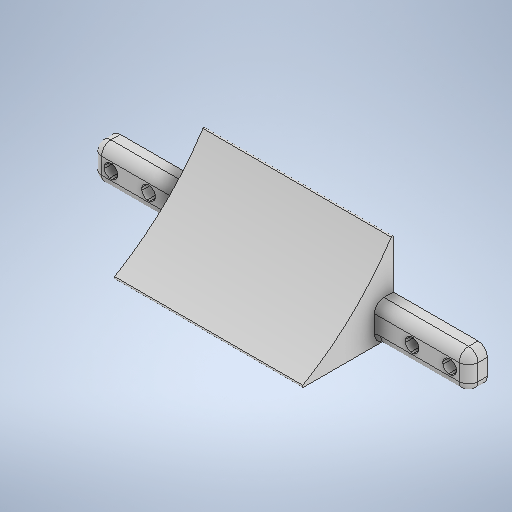
# Autodesk Inventor part: intake ramp piece
Saved by Autodesk Inventor 2025.1 (Build 291241020, 241B)
## iProperties
Created: 2024-12-04
Part Number: intake ramp piece
Material: Generic
Document SubType Name: Modeling
Designer: Hunter Mathis
Density: 1 g/cm^3
Appearance: Default
Author: Hunter Mathis
Autodesk Inventor part; units mm, degrees
ref_plane "YZ Plane" through (0, 0, 0) normal (1, 0, 0) x (0, 1, 0)
ref_plane "XZ Plane" through (0, 0, 0) normal (0, 1, 0) x (-1, 0, 0)
ref_plane "XY Plane" through (0, 0, 0) normal (0, 0, 1) x (1, 0, 0)
sketch "Sketch1" plane through (0, 0, 0) normal (0, 0, 1) x (1, 0, 0)
  line L0 (0, 0) -> (127, 0)
  line L1 (127, 0) -> (127, 11.9126)
  line L2 (127, 11.9126) -> (0, 11.9126)
  line L3 (0, 11.9126) -> (0, 0)
  dimension "d0" = 127
  dimension "d1" = 11.9126
  constraints: 8 end point, 2 parallel, 1 horizontal, 1 perpendicular
  measures "d0" distance of L1.end L2.end
  measures "d1" distance of L0.end L1.end
extrude "Extrusion1" add sketch "Sketch1" along normal blind 6.35
sketch "Sketch3" plane through (0, 0, 0) normal (0, 0, -1) x (-1, 0, 0)
  line L0 (-127, 0) -> (-127, 11.9126) projected
  line L1 (-127, 5.9563) -> (-120.65, 5.9563)
  line L2 (-127, 11.9126) -> (0, 11.9126) projected
  line L3 (0, 0) -> (-127, 0) projected
  line L4 (0, 11.9126) -> (0, 0) projected
  line L5 (-121.412, 8.2423) -> (-119.888, 8.2423)
  line L6 (-118.364, 6.7183) -> (-118.364, 5.1943)
  line L7 (-119.888, 3.6703) -> (-121.412, 3.6703)
  line L8 (-122.936, 5.1943) -> (-122.936, 6.7183)
  arc A0 (-121.412, 8.2423) -> (-122.936, 6.7183) centre (-121.412, 6.7183) ccw
  arc A1 (-118.364, 6.7183) -> (-119.888, 8.2423) centre (-119.888, 6.7183) ccw
  arc A2 (-119.888, 3.6703) -> (-118.364, 5.1943) centre (-119.888, 5.1943) ccw
  arc A3 (-122.936, 5.1943) -> (-121.412, 3.6703) centre (-121.412, 5.1943) ccw
  line L9 (-107.188, 3.6703) -> (-108.712, 3.6703)
  line L10 (-105.664, 6.7183) -> (-105.664, 5.1943)
  arc A4 (-105.664, 6.7183) -> (-107.188, 8.2423) centre (-107.188, 6.7183) ccw
  arc A5 (-110.236, 5.1943) -> (-108.712, 3.6703) centre (-108.712, 5.1943) ccw
  line L11 (-110.236, 5.1943) -> (-110.236, 6.7183)
  line L12 (-108.712, 8.2423) -> (-107.188, 8.2423)
  arc A6 (-108.712, 8.2423) -> (-110.236, 6.7183) centre (-108.712, 6.7183) ccw
  arc A7 (-107.188, 3.6703) -> (-105.664, 5.1943) centre (-107.188, 5.1943) ccw
  line L13 (-94.488, 3.6703) -> (-96.012, 3.6703)
  line L14 (-92.964, 6.7183) -> (-92.964, 5.1943)
  arc A8 (-92.964, 6.7183) -> (-94.488, 8.2423) centre (-94.488, 6.7183) ccw
  arc A9 (-97.536, 5.1943) -> (-96.012, 3.6703) centre (-96.012, 5.1943) ccw
  line L15 (-97.536, 5.1943) -> (-97.536, 6.7183)
  line L16 (-96.012, 8.2423) -> (-94.488, 8.2423)
  arc A10 (-96.012, 8.2423) -> (-97.536, 6.7183) centre (-96.012, 6.7183) ccw
  arc A11 (-94.488, 3.6703) -> (-92.964, 5.1943) centre (-94.488, 5.1943) ccw
  line L17 (-81.788, 3.6703) -> (-83.312, 3.6703)
  line L18 (-80.264, 6.7183) -> (-80.264, 5.1943)
  arc A12 (-80.264, 6.7183) -> (-81.788, 8.2423) centre (-81.788, 6.7183) ccw
  arc A13 (-84.836, 5.1943) -> (-83.312, 3.6703) centre (-83.312, 5.1943) ccw
  line L19 (-84.836, 5.1943) -> (-84.836, 6.7183)
  line L20 (-83.312, 8.2423) -> (-81.788, 8.2423)
  arc A14 (-83.312, 8.2423) -> (-84.836, 6.7183) centre (-83.312, 6.7183) ccw
  arc A15 (-81.788, 3.6703) -> (-80.264, 5.1943) centre (-81.788, 5.1943) ccw
  line L21 (-69.088, 3.6703) -> (-70.612, 3.6703)
  line L22 (-67.564, 6.7183) -> (-67.564, 5.1943)
  arc A16 (-67.564, 6.7183) -> (-69.088, 8.2423) centre (-69.088, 6.7183) ccw
  arc A17 (-72.136, 5.1943) -> (-70.612, 3.6703) centre (-70.612, 5.1943) ccw
  line L23 (-72.136, 5.1943) -> (-72.136, 6.7183)
  line L24 (-70.612, 8.2423) -> (-69.088, 8.2423)
  arc A18 (-70.612, 8.2423) -> (-72.136, 6.7183) centre (-70.612, 6.7183) ccw
  arc A19 (-69.088, 3.6703) -> (-67.564, 5.1943) centre (-69.088, 5.1943) ccw
  line L25 (-56.388, 3.6703) -> (-57.912, 3.6703)
  line L26 (-54.864, 6.7183) -> (-54.864, 5.1943)
  arc A20 (-54.864, 6.7183) -> (-56.388, 8.2423) centre (-56.388, 6.7183) ccw
  arc A21 (-59.436, 5.1943) -> (-57.912, 3.6703) centre (-57.912, 5.1943) ccw
  line L27 (-59.436, 5.1943) -> (-59.436, 6.7183)
  line L28 (-57.912, 8.2423) -> (-56.388, 8.2423)
  arc A22 (-57.912, 8.2423) -> (-59.436, 6.7183) centre (-57.912, 6.7183) ccw
  arc A23 (-56.388, 3.6703) -> (-54.864, 5.1943) centre (-56.388, 5.1943) ccw
  line L29 (-43.688, 3.6703) -> (-45.212, 3.6703)
  line L30 (-42.164, 6.7183) -> (-42.164, 5.1943)
  arc A24 (-42.164, 6.7183) -> (-43.688, 8.2423) centre (-43.688, 6.7183) ccw
  arc A25 (-46.736, 5.1943) -> (-45.212, 3.6703) centre (-45.212, 5.1943) ccw
  line L31 (-46.736, 5.1943) -> (-46.736, 6.7183)
  line L32 (-45.212, 8.2423) -> (-43.688, 8.2423)
  arc A26 (-45.212, 8.2423) -> (-46.736, 6.7183) centre (-45.212, 6.7183) ccw
  arc A27 (-43.688, 3.6703) -> (-42.164, 5.1943) centre (-43.688, 5.1943) ccw
  line L33 (-30.988, 3.6703) -> (-32.512, 3.6703)
  line L34 (-29.464, 6.7183) -> (-29.464, 5.1943)
  arc A28 (-29.464, 6.7183) -> (-30.988, 8.2423) centre (-30.988, 6.7183) ccw
  arc A29 (-34.036, 5.1943) -> (-32.512, 3.6703) centre (-32.512, 5.1943) ccw
  line L35 (-34.036, 5.1943) -> (-34.036, 6.7183)
  line L36 (-32.512, 8.2423) -> (-30.988, 8.2423)
  arc A30 (-32.512, 8.2423) -> (-34.036, 6.7183) centre (-32.512, 6.7183) ccw
  arc A31 (-30.988, 3.6703) -> (-29.464, 5.1943) centre (-30.988, 5.1943) ccw
  line L37 (-18.288, 3.6703) -> (-19.812, 3.6703)
  line L38 (-16.764, 6.7183) -> (-16.764, 5.1943)
  arc A32 (-16.764, 6.7183) -> (-18.288, 8.2423) centre (-18.288, 6.7183) ccw
  arc A33 (-21.336, 5.1943) -> (-19.812, 3.6703) centre (-19.812, 5.1943) ccw
  line L39 (-21.336, 5.1943) -> (-21.336, 6.7183)
  line L40 (-19.812, 8.2423) -> (-18.288, 8.2423)
  arc A34 (-19.812, 8.2423) -> (-21.336, 6.7183) centre (-19.812, 6.7183) ccw
  arc A35 (-18.288, 3.6703) -> (-16.764, 5.1943) centre (-18.288, 5.1943) ccw
  line L41 (-5.588, 3.6703) -> (-7.112, 3.6703)
  line L42 (-4.064, 6.7183) -> (-4.064, 5.1943)
  arc A36 (-4.064, 6.7183) -> (-5.588, 8.2423) centre (-5.588, 6.7183) ccw
  arc A37 (-8.636, 5.1943) -> (-7.112, 3.6703) centre (-7.112, 5.1943) ccw
  line L43 (-8.636, 5.1943) -> (-8.636, 6.7183)
  line L44 (-7.112, 8.2423) -> (-5.588, 8.2423)
  arc A38 (-7.112, 8.2423) -> (-8.636, 6.7183) centre (-7.112, 6.7183) ccw
  arc A39 (-5.588, 3.6703) -> (-4.064, 5.1943) centre (-5.588, 5.1943) ccw
  circle A40 centre (-120.65, 5.9563) radius 2.3241
  circle A41 centre (-107.95, 5.9563) radius 2.3241
  circle A42 centre (-19.05, 5.9563) radius 2.3241
  circle A43 centre (-6.35, 5.9563) radius 2.3241
  point P0 (-95.25, 5.9563)
  point P1 (-82.55, 5.9563)
  point P2 (-69.85, 5.9563)
  point P3 (-57.15, 5.9563)
  point P4 (-44.45, 5.9563)
  point P5 (-31.75, 5.9563)
  point P6 (-4.064, 6.3754)
  point P7 (-5.9309, 8.2423)
  point P8 (-6.7691, 8.2423)
  point P9 (-8.636, 6.3754)
  point P10 (-8.636, 5.5372)
  point P11 (-6.7691, 3.6703)
  point P12 (-5.9309, 3.6703)
  point P13 (-4.064, 5.5372)
  point P14 (-16.764, 6.3754)
  point P15 (-18.6309, 8.2423)
  point P16 (-19.4691, 8.2423)
  point P17 (-21.336, 6.3754)
  point P18 (-21.336, 5.5372)
  point P19 (-19.4691, 3.6703)
  point P20 (-18.6309, 3.6703)
  point P21 (-16.764, 5.5372)
  point P22 (-105.664, 6.3754)
  point P23 (-107.5309, 8.2423)
  point P24 (-108.3691, 8.2423)
  point P25 (-110.236, 6.3754)
  point P26 (-110.236, 5.5372)
  point P27 (-108.3691, 3.6703)
  point P28 (-107.5309, 3.6703)
  point P29 (-105.664, 5.5372)
  point P30 (-118.364, 6.3754)
  point P31 (-120.2309, 8.2423)
  point P32 (-121.0691, 8.2423)
  point P33 (-122.936, 6.3754)
  point P34 (-122.936, 5.5372)
  point P35 (-121.0691, 3.6703)
  point P36 (-120.2309, 3.6703)
  point P37 (-118.364, 5.5372)
  dimension "d9" = 6.35
  dimension "d31" = 1.524
  dimension "d34" = 12.7
  dimension "d39" = 4.6482
  dimension "d40" = 4.6482
  dimension "d41" = 4.6482
  dimension "d42" = 4.6482
  constraints: 82 end point, 80 point on circle, 44 centre point, 8 tangent, 4 coincident, 3 equal radius, 3 horizontal, 2 parallel, 1 midpoint, 1 perpendicular, 189 other
  measures "d9" distance of L1.end L1.start
  measures "d31" radius of A0
  measures "d34" distance of L1.end point (-107.95, 5.956)
  measures "d39" diameter of A40
  measures "d40" diameter of A41
  measures "d41" diameter of A42
  measures "d42" diameter of A43
extrude "Extrusion5" cut sketch "Sketch3" against normal through all contours L8 A40 L5 L6 L7 | L9 A41 L11 L12 L10 | L37 A42 L39 L40 L38 | L41 A43 L43 L44 L42
extrude "Extrusion6" add sketch "Sketch3" along normal blind 1.5875 contours L13 A9 L15 A10 L16 A8 L14 A11 | L17 A13 L19 A14 L20 A12 L18 A15 | L21 A17 L23 A18 L24 A16 L22 A19 | L25 A21 L27 A22 L28 A20 L26 A23 | L29 A25 L31 A26 L32 A24 L30 A27 | L33 A29 L35 A30 L36 A28 L34 A31
fillet "Fillet1" radius 3.175 4 edges at (0, 11.9126, 3.175) (0, 0, 3.175) (127, 0, 3.175) (127, 11.9126, 3.175)
sketch "Sketch5" plane through (0, 0, 6.35) normal (0, 0, 1) x (1, 0, 0)
  line L0 (0, 8.7376) -> (0, 3.175) projected
  line L1 (0, 5.9563) -> (63.5, 5.9563)
  line L2 (63.5, 5.9563) -> (63.5, 0)
  line L3 (3.175, 0) -> (123.825, 0) projected
  line L4 (95.25, -0.7937) -> (31.75, -0.7937)
  line L5 (31.75, -0.7937) -> (31.75, 0.7938)
  line L6 (31.75, 0.7938) -> (95.25, 0.7938)
  line L7 (95.25, 0.7938) -> (95.25, -0.7937)
  line L8 (95.25, -0.7937) -> (31.75, 0.7938) construction
  line L9 (31.75, -0.7937) -> (95.25, 0.7938) construction
  point P0 (0, 0)
  point P1 (95.25, 0)
  point P2 (31.75, 0)
  dimension "d49" = 63.5
  dimension "d50" = 63.5
  dimension "d57" = 1.5875
  constraints: 16 end point, 4 midpoint, 2 horizontal, 2 parallel, 1 perpendicular
  measures "d49" distance of L1.start L1.end
  measures "d50" distance of L5.end L6.end
  measures "d57" distance of L4.end L5.end
extrude "Extrusion7" add sketch "Sketch5" along normal blind 25.4
sketch "Sketch6" plane through (0, 0, 6.35) normal (0, 0, -1) x (-1, 0, 0)
  line L0 (-95.25, -0.7937) -> (-95.25, 0) projected
  line L1 (-95.25, 0) -> (-95.25, -0.7937)
  line L2 (-95.25, -0.7937) -> (-31.731, -0.7937)
  line L3 (-31.731, -0.7937) -> (-31.731, 0)
  line L4 (-31.731, 0) -> (-95.25, 0)
  point P0 (0, 0)
  constraints: 8 end point, 3 perpendicular, 1 vertical
extrude "Extrusion8" add sketch "Sketch6" along normal blind 6.35
sketch "Sketch7" plane through (31.75, 0.7938, 6.35) normal (0, 1, 0) x (1, 0, 0)
  line L0 (0, 0) -> (0, -25.4) projected
  line L1 (63.5, 0) -> (63.5, -25.4) projected
  line L2 (0, 0) -> (63.5, 0)
  line L3 (63.5, 0) -> (63.5, -25.4)
  line L4 (0, -25.4) -> (63.5, -25.4) projected
  line L5 (63.5, -25.4) -> (0, -25.4)
  line L6 (0, -25.4) -> (0, 0)
  point P0 (-31.75, 6.35)
  constraints: 8 end point, 2 collinear, 1 horizontal, 1 perpendicular
extrude "Extrusion9" add sketch "Sketch7" along normal blind 29.21
fillet "Fillet6" radius 3.175 1 edges at (31.731, 0, 3.175)
fillet "Fillet7" radius 3.175 1 edges at (95.25, 0, 3.175)
fillet "Fillet9" radius 3.175 5 edges at (0.9299, 10.9827, 6.35) (0, 5.9563, 6.35) (0.9299, 0.9299, 6.35) (16.403, 0, 6.35) (30.7535, -0.2051, 6.35)
fillet "Fillet11" radius 3.175 4 edges at (126.0701, 0.9299, 6.35) (127, 5.9563, 6.35) (96.2275, -0.2051, 6.35) (110.5875, 0, 6.35)
sketch "Sketch16" plane through (3.175, 11.9126, 0) normal (0, 1, 0) x (1, 0, 0)
  line L0 (92.075, -6.35) -> (28.575, -6.35) projected
  line L1 (92.075, -3.175) -> (92.075, 0) projected
  line L2 (92.075, -6.35) -> (92.075, 0)
  line L3 (92.075, 0) -> (27.6367, 0)
  line L4 (28.575, -6.35) -> (28.575, 0)
  line L5 (120.65, 0) -> (0, 0) projected
  line L6 (26.456, -6.35) -> (28.575, -6.35) projected
  line L7 (28.575, -6.35) -> (92.075, -6.35)
  point P0 (-3.175, 0)
  constraints: 8 end point, 2 collinear, 2 perpendicular, 1 point on line
extrude "Extrusion17" add sketch "Sketch16" along normal blind 17.4625
sketch "Sketch17" plane through (31.75, -0.7937, 31.75) normal (-1, 0, 0) x (0, 0, 1)
  line L0 (-31.75, 30.1688) -> (-25.4, 30.1688) projected
  line L1 (-28.2927, 0) -> (0, 0) projected
  arc A0 (-31.75, 30.1688) -> (0, 0) centre (43.4747, 77.5446) ccw
  line L2 (-31.75, 30.1688) -> (-31.75, 35.6548)
  line L3 (-31.75, 35.6548) -> (0, 35.6548)
  line L4 (0, 35.6548) -> (0, 0)
  point P0 (-31.75, 0.7937)
  dimension "d87" = 88.9
  constraints: 6 end point, 2 perpendicular, 2 point on circle, 1 centre point, 1 vertical
  measures "d87" radius of A0
extrude "Extrusion18" cut sketch "Sketch17" against normal through all
fillet "Fillet13" radius 0.381 1 edges at (63.5, 29.3751, 0)
fillet "Fillet14" radius 0.381 1 edges at (63.5, -0.7937, 31.75)
body "Solid1"
